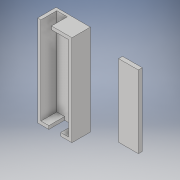
# Autodesk Inventor part: mcu_housing
Saved by Autodesk Inventor 2019 (Build 230136000, 136)
## iProperties
Created: 2024-04-30
Part Number: mcu_housing
Material: Generisch
Document SubType Name: Modeling
Designer: nic
Density: 1 g/cm^3
Appearance: Vorgabe
Author: nic
Autodesk Inventor part; units mm, degrees
ref_plane "YZ Plane" through (0, 0, 0) normal (1, 0, 0) x (0, 1, 0)
ref_plane "XZ Plane" through (0, 0, 0) normal (0, 1, 0) x (-1, 0, 0)
ref_plane "XY Plane" through (0, 0, 0) normal (0, 0, 1) x (1, 0, 0)
sketch "Skizze1" plane through (0, 0, 0) normal (0, 0, 1) x (1, 0, 0)
  line L0 (-10.5, 32) -> (10.5, 32)
  line L1 (10.5, 32) -> (10.5, -32)
  line L2 (10.5, -32) -> (-10.5, -32)
  line L3 (-10.5, -32) -> (-10.5, 32)
  line L4 (-10.5, 32) -> (10.5, -32) construction
  line L5 (10.5, 32) -> (-10.5, -32) construction
  line L6 (13, -34.5) -> (13, 34.5)
  line L7 (13, 34.5) -> (-13, 34.5)
  line L8 (-13, 34.5) -> (-13, -34.5)
  line L9 (-13, -34.5) -> (13, -34.5)
  point P0 (0, 0)
  dimension "d0" = 21
  dimension "d1" = 64
  dimension "d2" = 2.5
  constraints: 20 end point, 4 parallel, 2 midpoint, 2 perpendicular, 1 horizontal, 3 other
  measures "d0" distance of L1.end L2.end
  measures "d1" distance of L0.end L1.end
  measures "d2" distance between parallel lines of L1 L6
extrude "Extrusion1" add sketch "Skizze1" along normal blind 14
sketch "Skizze2" plane through (0, 0, 0) normal (0, 0, -1) x (-1, 0, 0)
  line L0 (-10.5, -32) -> (-10.5, 32) projected
  line L1 (-10.5, 32) -> (10.5, 32) projected
  line L2 (10.5, 32) -> (10.5, -32) projected
  line L3 (10.5, -32) -> (-10.5, -32) projected
  line L4 (-13, -34.5) -> (-13, 34.5) projected
  line L5 (13, -34.5) -> (-13, -34.5) projected
  line L6 (13, 34.5) -> (13, -34.5) projected
  line L7 (-13, 34.5) -> (13, 34.5) projected
  point P0 (0, 0)
extrude "Extrusion2" add sketch "Skizze2" against normal blind 2 contours L0 L1 L2 L3
sketch "Skizze3" plane through (-10.5, -32, 14) normal (0, 1, 0) x (1, 0, 0)
  line L0 (21, 12) -> (0, 12) projected
  line L1 (0, 12) -> (0, 0) projected
  line L2 (21, 0) -> (0, 0) projected
  line L3 (21, 12) -> (21, 0) projected
  line L4 (15, 27.4214) -> (6, 27.4214)
  line L5 (6, 27.4214) -> (6, -3.4214)
  line L6 (6, -3.4214) -> (15, -3.4214)
  line L7 (15, -3.4214) -> (15, 27.4214)
  line L8 (21, 12) -> (0, 12) projected
  line L9 (15, 27.4214) -> (6, -3.4214) construction
  line L10 (6, 27.4214) -> (15, -3.4214) construction
  line L11 (15, 12) -> (6, 12)
  point P0 (10.5, 14)
  point P1 (10.5, 12)
  dimension "d7" = 9
  constraints: 14 end point, 5 midpoint, 2 parallel, 2 point on line, 1 horizontal, 1 perpendicular
  measures "d7" distance of L6.end L5.end
extrude "Extrusion3" cut sketch "Skizze3" against normal through all contours L7 L2 L5 L0 | L7 L6 L5 L2
sketch "Skizze4" plane through (0, 0, 14) normal (0, 0, 1) x (1, 0, 0)
  line L0 (-10.5, 32) -> (10.5, 32) projected
  line L1 (13, 34.5) -> (-13, 34.5) projected
  line L2 (-10.5, 32) -> (-2.5, 32)
  line L3 (-2.5, 32) -> (-2.5, 34.5)
  line L4 (-2.5, 34.5) -> (-10.5, 34.5)
  line L5 (-10.5, 34.5) -> (-10.5, 32)
  point P0 (0, 0)
  dimension "d10" = 8
  constraints: 8 end point, 2 parallel, 1 horizontal, 1 perpendicular, 1 point on line
  measures "d10" distance of L4.end L3.end
extrude "Extrusion4" cut sketch "Skizze4" against normal up to surface (12 mm away)
sketch "Skizze5" plane through (0, 0, 0) normal (0, 0, 1) x (1, 0, 0)
  line L0 (37.4447, -27.5) -> (52.4447, -27.5)
  line L1 (52.4447, -27.5) -> (52.4447, 27.5)
  line L2 (52.4447, 27.5) -> (37.4447, 27.5)
  line L3 (37.4447, 27.5) -> (37.4447, -27.5)
  line L4 (37.4447, -27.5) -> (52.4447, 27.5) construction
  line L5 (52.4447, -27.5) -> (37.4447, 27.5) construction
  point P0 (0, 0)
  point P1 (44.9447, 0)
  dimension "d13" = 15
  dimension "d14" = 55
  constraints: 12 end point, 2 midpoint, 2 parallel, 1 horizontal, 1 perpendicular
  measures "d13" distance of L2.end L1.end
  measures "d14" distance of L1.end L0.end
extrude "Extrusion5" add sketch "Skizze5" along normal blind 3
